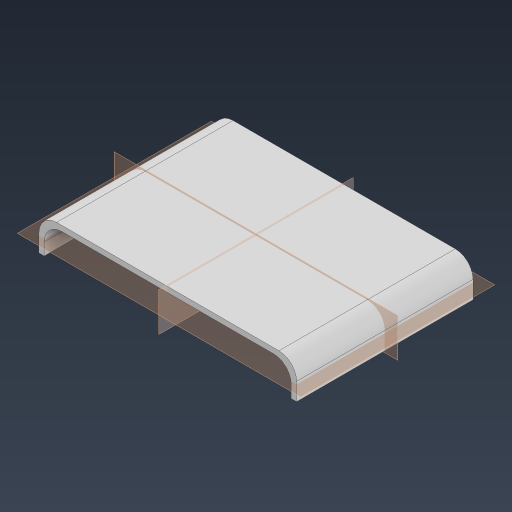
# Autodesk Inventor part: Крышка_электроники
Saved by Autodesk Inventor 2023.2 (Build 272271030, 271C)
## iProperties
Created: 2025-12-29
Part Number: Крышка_электроники
Material: Типовые
Document SubType Name: Modeling
Designer: Олег Коноваленко
Density: 1 g/cm^3
Appearance: По умолчанию
Author: Олег Коноваленко
Autodesk Inventor part; units mm, degrees
sketch "Эскиз1" plane through (0, 0, 0) normal (0, 0, 1) x (1, 0, 0)
  line L0 (-73, -8.5) -> (-73, 11.5)
  line L1 (-73, 11.5) -> (73, 11.5)
  line L2 (73, 11.5) -> (73, -8.5)
  line L3 (73, -8.5) -> (70, -8.5)
  line L4 (70, -8.5) -> (70, 8.5)
  line L5 (70, 8.5) -> (-70, 8.5)
  line L6 (-70, 8.5) -> (-70, -8.5)
  line L7 (-70, -8.5) -> (-73, -8.5)
  line L8 (0, 15.5) -> (0, -12.5) construction
  line L9 (-102.2, 0) -> (102.2, 0) projected
  point P0 (0, 0)
  point P1 (0, 11.5)
  point P2 (-70, 0)
  dimension "d0" = 140
  dimension "d2" = 3
  dimension "d3" = 3
  dimension "d4" = 20
  constraints: 16 end point, 6 perpendicular, 2 equal length, 2 midpoint, 2 point on line, 1 parallel, 1 vertical
  measures "d0" distance between parallel lines of L4 L6
  measures "d2" distance between parallel lines of L5 L1
  measures "d3" distance between parallel lines of L2 L4
  measures "d4" distance of L0.start L0.end
extrude "Выдавливание1" add sketch "Эскиз1" along normal mid plane 100 contours L0 L9 L6 L7 | L0 L1 L2 L9 L4 L5 L6 | L9 L2 L3 L4
fillet "Сопряжение1" radius 10 4 edges at (-73, 11.5, 0) (-70, 8.5, 0) (70, 8.5, 0) (73, 11.5, 0)
